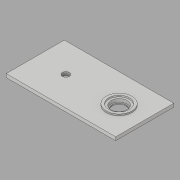
# Autodesk Inventor part: b_base cover_test 1
Saved by Autodesk Inventor 2019 (Build 230136000, 136)
## iProperties
Created: 2021-11-06
Part Number: b_base cover_test 1
Material: Generic
Document SubType Name: Modeling
Designer: Mohamed
Density: 1 g/cm^3
Appearance: Default
Author: Mohamed
Autodesk Inventor part; units mm, degrees
ref_plane "YZ Plane" through (0, 0, 0) normal (1, 0, 0) x (0, 1, 0)
ref_plane "XZ Plane" through (0, 0, 0) normal (0, 1, 0) x (-1, 0, 0)
ref_plane "XY Plane" through (0, 0, 0) normal (0, 0, 1) x (1, 0, 0)
sketch "Sketch1" plane through (0, 0, 0) normal (0, 1, 0) x (-1, 0, 0)
  line L0 (0, 0) -> (250, 0)
  line L1 (250, 0) -> (250, -170)
  line L2 (250, -170) -> (0, -170)
  line L3 (0, -170) -> (0, 0)
  line L4 (0, 0) -> (150, 0)
  dimension "d0" = 250
  dimension "d1" = 170
  dimension "d2" = 150
  constraints: 10 end point, 2 parallel, 1 horizontal, 1 perpendicular, 1 point on line
  measures "d0" distance of L1.end L2.end
  measures "d1" distance of L0.end L1.end
  measures "d2" distance of L0.start L4.end
extrude "Extrusion1" add sketch "Sketch1" along normal blind 10
sketch "Sketch2" plane through (0, 10, 0) normal (0, 1, 0) x (1, 0, 0)
  line L0 (0, 0) -> (-150, 0)
  line L1 (-250, 0) -> (0, 0) projected
  line L2 (0, 170) -> (-250, 170) projected
  circle A0 centre (-75, 85) radius 20
  dimension "d5" = 150
  dimension "d6" = 40
  constraints: 2 end point, 1 centre point, 1 point on line
  measures "d5" distance of L0.start L0.end
  measures "d6" diameter of A0
extrude "Extrusion2" cut sketch "Sketch2" against normal blind 10
sketch "Sketch3" plane through (0, 10, 0) normal (0, 1, 0) x (1, 0, 0)
  circle A0 centre (-75, 85) radius 20 projected
  circle A1 centre (-75, 85) radius 23.5
  point P0 (0, 0)
  dimension "d9" = 47
  constraints: 1 centre point, 1 coincident
  measures "d9" diameter of A1
extrude "Extrusion3" cut sketch "Sketch3" against normal blind 9
sketch "Sketch4" plane through (0, 10, 0) normal (0, 1, 0) x (1, 0, 0)
  circle A0 centre (-75, 85) radius 20 projected
  circle A1 centre (-75, 85) radius 30
  circle A2 centre (-75, 85) radius 37.5
  point P0 (0, 0)
  dimension "d12" = 60
  dimension "d13" = 75
  constraints: 2 centre point, 2 coincident
  measures "d12" diameter of A1
  measures "d13" diameter of A2
extrude "Extrusion4" add sketch "Sketch4" along normal blind 4 contours A2
sketch "Sketch5" plane through (0, 0, 0) normal (0, -1, 0) x (1, 0, 0)
  circle A0 centre (-75, -85) radius 20 projected
  circle A1 centre (-75, -85) radius 20.5
  circle A2 centre (-75, -85) radius 20
  point P0 (0, 0)
  dimension "d16" = 41
  dimension "d17" = 40
  constraints: 2 centre point, 2 coincident
  measures "d16" diameter of A1
  measures "d17" diameter of A2
extrude "Extrusion5" add sketch "Sketch5" along normal blind 2
sketch "Sketch6" plane through (0, 10, 0) normal (0, 1, 0) x (1, 0, 0)
  circle A0 centre (-75, 85) radius 23.5 projected
  circle A1 centre (-75, 85) radius 50
  circle A2 centre (-230.6, 85) radius 10
  point P0 (0, 0)
  dimension "d20" = 100
  dimension "d22" = 20
  constraints: 2 centre point, 1 coincident
  measures "d20" diameter of A1
  measures "d22" diameter of A2
extrude "Extrusion6" cut sketch "Sketch6" against normal blind 10 contours A2
sketch "Sketch7" plane through (0, 0, 0) normal (0, -1, 0) x (1, 0, 0)
  line L0 (-250, -170) -> (-250, 0) projected
  line L1 (-250, 0) -> (-320, 0)
  line L2 (-320, 0) -> (-320, -170)
  line L3 (-320, -170) -> (-250, -170)
  line L4 (-250, -170) -> (-250, 0)
  point P0 (0, 0)
  dimension "d25" = 70
  dimension "d26" = 170
  constraints: 8 end point, 2 parallel, 1 horizontal, 1 perpendicular
  measures "d25" distance of L3.end L2.end
  measures "d26" distance of L2.end L1.end
extrude "Extrusion7" add sketch "Sketch7" against normal blind 10
body "Solid1"
